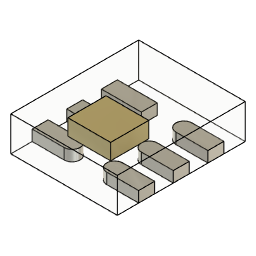
AMS_TSL2591 (Autodesk Fusion 360 design; units mm, degrees)
Autodesk Fusion 360 part; units mm, degrees
sketch "Sketch1" plane through (0, 0, 0) normal (0, 0, 1) x (1, 0, 0) in component "Body"
  line L0 (1, -1.2) -> (-1, -1.2)
  line L1 (-1, -1.2) -> (-1, 1.2)
  line L2 (-1, 1.2) -> (1, 1.2)
  line L3 (1, 1.2) -> (1, -1.2)
  line L4 (1, -1.2) -> (-1, 1.2) construction
  line L5 (-1, -1.2) -> (1, 1.2) construction
  dimension "d1" = 2
  dimension "d2" = 2.4
  constraint horizontal L0
  constraint perpendicular L0 L1
  constraint parallel L0 L2
  constraint parallel L1 L3
  constraint coincident L4 origin
  constraint coincident L5 origin
  measures "d1" distance of L1.end L2.end
  measures "d2" distance of L0.end L1.end
extrude "Extrude1" add sketch "Sketch1" along normal blind 0.65 makes body 1 in component "Body"
sketch "Sketch3" plane through (0, 0, 0) normal (0, 0, -1) x (1, 0, 0) in component "Body"
  line L0 (-1, -1.2) -> (1, -1.2)
  line L1 (1, -1.2) -> (1, 1.2)
  line L2 (1, 1.2) -> (-1, 1.2)
  line L3 (-1, 1.2) -> (-1, -1.2)
  line L4 (-1, 0) -> (1, 0) construction
  line L5 (-1, 0.15) -> (-1, -0.15)
  line L6 (-1, 0.15) -> (-0.4, 0.15)
  line L7 (-1, -0.15) -> (-0.4, -0.15)
  line L8 (-0.25, 1.2) -> (-0.25, -1.2) construction
  line L9 (0.25, 1.2) -> (0.25, 1.1)
  line L10 (0.25, 1.1) -> (0.25, -1.2) construction
  line L11 (1, -0.15) -> (1, 0.15)
  line L12 (1, 0.15) -> (0.4, 0.15)
  line L13 (1, -0.15) -> (0.9731, -0.15)
  line L14 (0.9731, -0.15) -> (0.4, -0.15)
  arc A0 (0.4, 0.15) -> (0.4, -0.15) centre (0.4, 0) ccw
  arc A1 (-0.4, -0.15) -> (-0.4, 0.15) centre (-0.4, 0) ccw
  line L15 (-1, 0.65) -> (1, 0.65) construction
  line L16 (-1, -0.65) -> (1, -0.65) construction
  line L17 (1, 0.8) -> (1, 0.5)
  line L18 (1, -0.5) -> (1, -0.8)
  line L19 (-1, 0.8) -> (-1, 0.5)
  line L20 (-1, -0.5) -> (-1, -0.8)
  line L21 (1, 0.8) -> (0.9979, 0.8)
  line L22 (0.9979, 0.8) -> (0.4, 0.8)
  line L23 (1, -0.5) -> (0.4, -0.5)
  line L24 (-1, 0.8) -> (-0.4, 0.8)
  line L25 (-1, 0.5) -> (-0.4, 0.5)
  arc A2 (-0.4, 0.5) -> (-0.4, 0.8) centre (-0.4, 0.65) ccw
  arc A3 (0.4, 0.8) -> (0.401, 0.5) centre (0.4, 0.65) ccw
  arc A4 (0.4, -0.5) -> (0.4, -0.8) centre (0.4, -0.65) ccw
  line L26 (0.4, -0.8) -> (1, -0.8)
  line L27 (-1, -0.5) -> (-0.25, -0.5)
  line L28 (-1, -0.8) -> (-0.25, -0.8)
  line L29 (-0.25, -0.8) -> (-0.25, -0.5)
  line L30 (0.401, 0.5) -> (1, 0.5)
  dimension "d13" = 0.3
  dimension "d16" = 0.75
  dimension "d18" = 0.75
  dimension "d19" = 0.3
  dimension "d20" = 0.15
  dimension "d21" = 0.65
  dimension "d22" = 0.65
  dimension "d23" = 0.6
  dimension "d24" = 0.6
  dimension "d25" = 0.6
  dimension "d26" = 0.6
  constraint midpoint L3 L4.start
  constraint midpoint L1 L4.end
  constraint coincident L3 L5.start
  constraint coincident L3 L5.end
  constraint parallel L3 L5
  constraint symmetric L4 L5.start L5.end
  constraint perpendicular L5 L6
  constraint perpendicular L5 L7
  constraint equal L6 L7
  constraint coincident L2 L8.start
  constraint coincident L0 L8.end
  constraint perpendicular L0 L8
  constraint coincident L2 L9.start
  constraint perpendicular L2 L9
  constraint coincident L0 L10.end
  constraint perpendicular L0 L10
  constraint coincident L1 L11.start
  constraint coincident L1 L11.end
  constraint parallel L1 L11
  constraint symmetric L4 L11.start L11.end
  constraint perpendicular L11 L12
  constraint perpendicular L1 L13
  constraint perpendicular L1 L14
  constraint coincident L4 A0.centre
  constraint tangent L10 A0
  constraint coincident L4 A1.centre
  constraint tangent L8 A1
  constraint coincident L1 L15.end
  constraint perpendicular L1 L15
  constraint coincident L3 L16.start
  constraint coincident L1 L16.end
  constraint perpendicular L3 L16
  constraint coincident L1 L17.start
  constraint coincident L1 L17.end
  constraint parallel L1 L17
  constraint coincident L1 L18.start
  constraint coincident L1 L18.end
  constraint perpendicular L16 L18
  constraint coincident L3 L19.start
  constraint coincident L3 L19.end
  constraint parallel L3 L19
  constraint coincident L3 L20.start
  constraint coincident L3 L20.end
  constraint perpendicular L4 L20
  constraint symmetric L15 L19.start L19.end
  constraint symmetric L15 L17.start L17.end
  constraint symmetric L16 L18.start L18.end
  constraint symmetric L16 L20.start L20.end
  constraint coincident L15.start L19
  constraint equal L17 L19
  constraint equal L17 L18
  constraint equal L18 L20
  constraint equal L5 L20
  constraint perpendicular L17 L21
  constraint perpendicular L17 L22
  constraint perpendicular L18 L23
  constraint perpendicular L3 L24
  constraint perpendicular L19 L25
  constraint equal L24 L25
  constraint coincident L15 A2.centre
  constraint coincident L15 A3.centre
  constraint coincident L16 A4.centre
  constraint tangent L10 A3
  constraint tangent L10 A4
  constraint tangent L8 A2
  constraint perpendicular L18 L26
  constraint equal L23 L26
  constraint coincident L8 L27.end
  constraint perpendicular L8 L27
  constraint coincident L8 L28.end
  constraint perpendicular L8 L28
  measures "d13" distance of L5.start L5.end
  measures "d16" distance of L2.end L8.start
  measures "d18" distance of L1.end L9.start
  measures "d19" distance of L11.start L11.end
  measures "d20" radius of A1
  measures "d21" distance of L4.end L15.end
  measures "d22" distance of L4.end L16.end
  measures "d23" distance of L11.end L12.end
  measures "d24" distance of L17.start L22.end
  measures "d25" distance of L18.start L23.end
  measures "d26" distance of L19.start L24.end
extrude "Extrude3" cut sketch "Sketch3" against normal blind 0.203 contours L3 L20 L27 L28 L29 | L1 L18 L23 A4 L26 | L3 L5 L6 L7 A1 | L1 L11 L12 L13 L14 A0 | L3 L19 L24 L25 A2 | L1 L17 L21 L22 A3 L30 bodies 1 in component "Body"
extrude "Extrude1'" add 6 faces at (-0.6, -0.6, 0.203) (0.6003, -0.7, 0.203) (0.8, 0.05, 0.203) (-0.6, 0.05, 0.203) (-0.5, 0.7, 0.203) (0.8, 0.7, 0.203) along direction (0, 0, -1) up to surface separate body end surface through (0, 0, 0) normal (0, 0, -1) offset 0 on bodies 1 makes body 2 at (-0.5, 0.7, 0.203) makes body 3 at (0.8, 0.05, 0.203) makes body 4 at (-0.6, -0.6, 0.203) makes body 5 at (0.6003, -0.7, 0.203) makes body 6 at (-0.6, 0.05, 0.203) makes body 7 at (0.8, 0.7, 0.203) in component "Pads"
sketch "Sketch4" plane through (0, 0, 0.65) normal (0, 0, 1) x (-1, 0, 0) in component "Body"
  line L0 (-1, -1.2) -> (1, -1.2)
  line L1 (1, -1.2) -> (1, 1.2)
  line L2 (1, 1.2) -> (-1, 1.2)
  line L3 (-1, 1.2) -> (-1, -1.2)
  line L4 (0, -1.2) -> (0, 1.2) construction
  line L5 (1, 0) -> (-1, 0) construction
  line L6 (-0.401, 0.728) -> (0.401, 0.728)
  line L7 (0.401, 0.728) -> (0.401, 0.012)
  line L8 (0.401, 0.012) -> (-0.401, 0.012)
  line L9 (-0.401, 0.012) -> (-0.401, 0.728)
  line L10 (-0.401, 0.728) -> (0.401, 0.012) construction
  line L11 (0.401, 0.728) -> (-0.401, 0.012) construction
  point P0 (0, 0.37)
  dimension "d50" = 0.802
  dimension "d51" = 0.716
  dimension "d52" = 0.37
  constraint midpoint L0 L4.start
  constraint midpoint L2 L4.end
  constraint midpoint L1 L5.start
  constraint midpoint L3 L5.end
  constraint horizontal L6
  constraint perpendicular L6 L7
  constraint parallel L6 L8
  constraint parallel L7 L9
  constraint coincident L10 P0
  constraint coincident L11 P0
  constraint coincident L4 P0
  measures "d50" distance of L7.end L8.end
  measures "d51" distance of L6.end L7.end
  measures "d52" distance of L5 P0
extrude "Extrude4" cut sketch "Sketch4" against normal blind 0.3 contours L6 L7 L8 L9 bodies 1 in component "Body"
extrude "Extrude7" add 1 faces at (0.1337, -0.4893, 0.35) along direction (0, 0, 1) up to surface (0.3 mm away) separate body on bodies 1 makes body 8 in component "Photodiode"
component "Body" placed x (1, 0, 0) y (0, 1, 0) z (0, 0, 1) at (0, 0, 0)
component "Photodiode" placed x (1, 0, 0) y (0, 1, 0) z (0, 0, 1) at (0, 0, 0)
component "Pads" placed x (1, 0, 0) y (0, 1, 0) z (0, 0, 1) at (0, 0, 0)
equation "d18 = d16"
equation "d19 = d13"
equation "d22 = d21"
equation "d24 = d23"
equation "d25 = d23"
equation "d26 = d23"
equation "d35 = 0.369 mm / 3"
equation "d36 = 0.406 mm / 4"
equation "d37 = d36"
